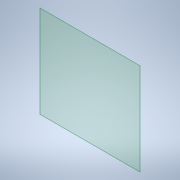
# Autodesk Inventor part: side panel
Saved by Autodesk Inventor 2020.4 (Build 244396000, 396)
## iProperties
Created: 2021-04-06
Part Number: side panel
Material: Glass
Document SubType Name: Modeling
Designer: AOB
Mass: 998.08 g
Surface Area: 5802.13 cm^2
Volume: 457.835 cm^3
Density: 2.18 g/cm^3
Appearance: Clear - Green 1
Author: AOB
Autodesk Inventor part; units mm, degrees
ref_plane "YZ Plane" through (0, 0, 0) normal (1, 0, 0) x (0, 1, 0)
ref_plane "XZ Plane" through (0, 0, 0) normal (0, 1, 0) x (-1, 0, 0)
ref_plane "XY Plane" through (0, 0, 0) normal (0, 0, 1) x (1, 0, 0)
sketch "Sketch1" plane through (0, 0, 0) normal (0, 0, 1) x (1, 0, 0)
  line L0 (0, 0) -> (560, 0)
  line L1 (560, 0) -> (560, -515)
  line L2 (560, -515) -> (0, -515)
  line L3 (0, -515) -> (0, 0)
  dimension "d0" = 560
  dimension "d1" = 515
  constraints: 8 end point, 2 parallel, 1 horizontal, 1 perpendicular
  measures "d0" distance of L1.end L2.end
  measures "d1" distance of L0.end L1.end
extrude "Extrusion1" add sketch "Sketch1" along normal blind 1.5875
body "Solid1"
